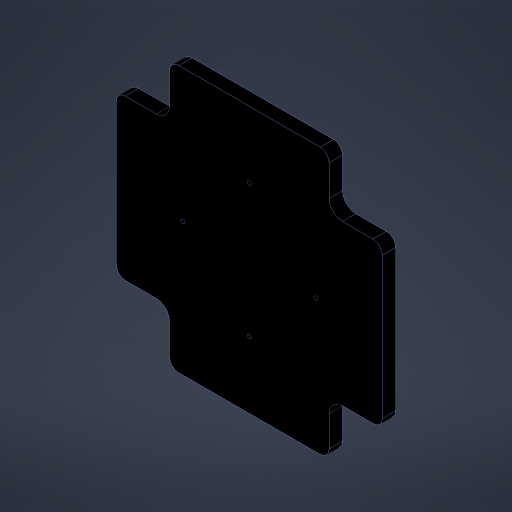
# Autodesk Inventor part: Base Motor
Saved by Autodesk Inventor 2023 (Build 270158000, 158)
## iProperties
Created: 2023-04-05
Part Number: Base Motor
Material: Aluminum 6061
Document SubType Name: Modeling
Designer: vatdu
Density: 2.7 g/cm^3
Appearance: Midnight Aluminum
Author: vatdu
Autodesk Inventor part; units mm, degrees
ref_plane "YZ Plane" through (0, 0, 0) normal (1, 0, 0) x (0, 1, 0)
ref_plane "XZ Plane" through (0, 0, 0) normal (0, 1, 0) x (-1, 0, 0)
ref_plane "XY Plane" through (0, 0, 0) normal (0, 0, 1) x (1, 0, 0)
sketch "Sketch1" plane through (0, 0, 0) normal (0, 0, 1) x (1, 0, 0)
  line L0 (0, 0) -> (200, 0)
  line L1 (200, 0) -> (200, 200)
  line L2 (200, 200) -> (0, 200)
  line L3 (0, 200) -> (0, 0)
  line L4 (0, 200) -> (40, 200)
  line L5 (40, 200) -> (40, 160)
  line L6 (40, 160) -> (0, 160)
  line L7 (0, 160) -> (0, 200)
  line L8 (200, 200) -> (160, 200)
  line L9 (160, 200) -> (160, 160)
  line L10 (160, 160) -> (200, 160)
  line L11 (200, 160) -> (200, 200)
  line L12 (200, 0) -> (160, 0)
  line L13 (160, 0) -> (160, 40)
  line L14 (160, 40) -> (200, 40)
  line L15 (200, 40) -> (200, 0)
  line L16 (0, 0) -> (40, 0)
  line L17 (40, 0) -> (40, 40)
  line L18 (40, 40) -> (0, 40)
  line L19 (0, 40) -> (0, 0)
  circle A0 centre (150, 100) radius 1.5
  circle A1 centre (50, 100) radius 1.5
  circle A2 centre (100, 150) radius 1.5
  circle A3 centre (100, 50.0402) radius 1.5
  point P0 (0, 40)
  point P1 (40, 0)
  point P2 (160, 0)
  point P3 (200, 40)
  point P4 (0, 160)
  dimension "d0" = 200
  dimension "d1" = 200
  dimension "d2" = 40
  dimension "d3" = 40
  dimension "d4" = 40
  dimension "d5" = 40
  dimension "d6" = 40
  dimension "d7" = 40
  dimension "d8" = 40
  dimension "d9" = 40
  dimension "d133" = 3
  dimension "d135" = 3
  dimension "d136" = 3
  dimension "d138" = 3
  constraints: 40 end point, 10 parallel, 5 horizontal, 5 perpendicular, 4 centre point
  measures "d0" distance of L2.end L1.end
  measures "d1" distance of L1.end L0.end
  measures "d2" distance of L5.end L6.end
  measures "d3" distance of L4.end L5.end
  measures "d4" distance of L10.end L9.end
  measures "d5" distance of L9.end L8.end
  measures "d6" distance of L13.end L14.end
  measures "d7" distance of L12.end L13.end
  measures "d8" distance of L18.end L17.end
  measures "d9" distance of L17.end L16.end
  measures "d133" diameter of A0
  measures "d135" diameter of A1
  measures "d136" diameter of A2
  measures "d138" diameter of A3
extrude "Extrusion1" add sketch "Sketch1" along normal blind 10 contours L17 L18 L3 L6 L5 L2 L9 L10 L1 L14 L13 L0
fillet "Fillet1" radius 10 4 edges at (160, 160, 5) (160, 40, 5) (40, 40, 5) (40, 160, 5)
fillet "Fillet2" radius 7 4 edges at (40, 200, 5) (200, 160, 5) (160, 0, 5) (0, 40, 5)
fillet "Fillet3" radius 6.735 4 edges at (40, 0, 5) (200, 40, 5) (0, 160, 5) (160, 200, 5)
scale "Scale2" factors (1.5, 1.5, 1.5) then translate (-50, -50, 0) bodies 1
body "Solid1"
